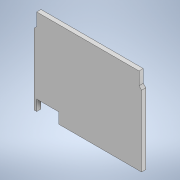
# Autodesk Inventor part: eonPCBcover
Saved by Autodesk Inventor 2020 (Build 240168000, 168)
## iProperties
Created: 2021-04-25
Part Number: eonPCBcover
Material: Generic
Document SubType Name: Modeling
Designer: dkiiv
Density: 1 g/cm^3
Appearance: Default
Author: dkiiv
Autodesk Inventor part; units mm, degrees
ref_plane "YZ Plane" through (0, 0, 0) normal (1, 0, 0) x (0, 1, 0)
ref_plane "XZ Plane" through (0, 0, 0) normal (0, 1, 0) x (-1, 0, 0)
ref_plane "XY Plane" through (0, 0, 0) normal (0, 0, 1) x (1, 0, 0)
sketch "Sketch1" plane through (0, 0, 0) normal (0, 0, 1) x (1, 0, 0)
  line L0 (0, 0) -> (42, 0)
  line L1 (42, 0) -> (42, 27.724)
  line L2 (0, 27.724) -> (0, 27.724)
  line L3 (0, 27.724) -> (0, 0)
  line L4 (1, 27.724) -> (41, 27.724)
  line L5 (41, 28.724) -> (41, 33.724)
  line L6 (41, 33.724) -> (1, 33.724)
  line L7 (1, 33.724) -> (1, 28.724)
  line L8 (1, 28.724) -> (0, 27.724)
  line L9 (42, 27.724) -> (42, 27.724)
  line L10 (41, 28.724) -> (42, 27.724)
  point P0 (1, 27.724)
  dimension "d0" = 27.724
  dimension "d1" = 42
  dimension "d2" = 0
  dimension "d3" = 40
  dimension "d4" = 1
  dimension "d5" = 1
  dimension "d6" = 1
  dimension "d7" = 1
  dimension "d8" = 1
  dimension "d9" = 5
  constraints: 22 end point, 6 point on line, 4 parallel, 2 horizontal, 2 perpendicular
  measures "d0" distance of L2.end L0.start
  measures "d1" distance of L0.start L0.end
  measures "d2" distance between parallel lines of L2 L4
  measures "d3" distance of L5.end L6.end
  measures "d4" distance between parallel lines of L3 L7
  measures "d5" distance of L7.end point (1, 27.724)
  measures "d6" distance of L2.start point (1, 27.724)
  measures "d7" distance of L5.start L4.end
  measures "d8" distance of L9.start L4.end
  measures "d9" distance of L5.start L5.end
extrude "Extrusion1" add sketch "Sketch1" along normal blind 1.667
sketch "Sketch2" plane through (0, 0, 1.667) normal (0, 0, 1) x (1, 0, 0)
  line L0 (32.3, 4.2) -> (41, 4.2)
  line L1 (41, 4.2) -> (41, 0)
  line L2 (41, 0) -> (32.3, 0)
  line L3 (32.3, 0) -> (32.3, 4.2)
  line L4 (0, 0) -> (42, 0) projected
  line L5 (1, 33.724) -> (1, 28.724) projected
  line L6 (41, 28.724) -> (41, 33.724) projected
  dimension "d12" = 0
  dimension "d14" = 8.7
  dimension "d15" = 4.2
  dimension "d18" = 0
  constraints: 8 end point, 2 parallel, 1 horizontal, 1 perpendicular
  measures "d12" distance between parallel lines of L4 L2
  measures "d14" distance of L0.start L0.end
  measures "d15" distance of L0.end L1.end
  measures "d18" distance between parallel lines of L6 L1
extrude "Extrusion2" cut sketch "Sketch2" against normal blind 2.083
equation "\"d6\" = d5"
equation "\"d8\" = d7"
body "Solid1"
